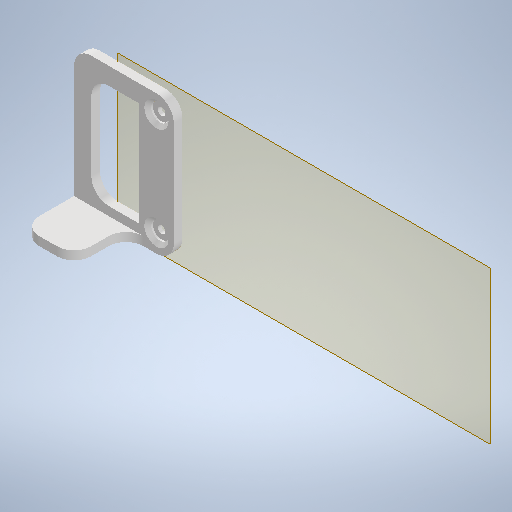
# Autodesk Inventor part: led 7 seg v3_stand
Saved by Autodesk Inventor 2026 (Build 300175000, 175)
## iProperties
Created: 2025-07-07
Part Number: led 7 seg v3_stand
Material: Generic
Document SubType Name: Modeling
Designer: Korobeynikov
Density: 1 g/cm^3
Appearance: Default
Author: Korobeynikov
Autodesk Inventor part; units mm, degrees
ref_plane "YZ Plane" through (0, 0, 0) normal (1, 0, 0) x (0, 1, 0)
ref_plane "XZ Plane" through (0, 0, 0) normal (0, 1, 0) x (-1, 0, 0)
ref_plane "XY Plane" through (0, 0, 0) normal (0, 0, 1) x (1, 0, 0)
ref_plane "Work Plane1" through (0, 0, 0) normal (0, 0, 1) x (1, 0, 0)
sketch "Sketch1" plane through (0, 0, 0) normal (0, 0, 1) x (1, 0, 0)
  circle A0 centre (-80, 29.5) radius 2.15 projected
  circle A1 centre (-80, -29.5) radius 2.15 projected
  line L0 (-127.5, 40) -> (-70, 40)
  line L1 (-70, 40) -> (-70, -40)
  line L2 (-70, -40) -> (-127.5, -40)
  line L3 (-127.5, -40) -> (-127.5, 40)
  line L4 (87.5, 40) -> (-87.5, 40) projected
  line L5 (-87.5, -40) -> (87.5, -40) projected
  line L6 (-97.5, 30) -> (-97.5, -30) projected
  line L7 (-117.5, 30) -> (-90, 30)
  line L8 (-90, 30) -> (-90, -30)
  line L9 (-90, -30) -> (-117.5, -30)
  line L10 (-117.5, -30) -> (-117.5, 30)
  point P0 (0, 0)
  point P1 (-117.5, 0)
  point P2 (-127.5, 0)
  dimension "d0" = 10
  dimension "d1" = 30
  dimension "d2" = 10
  dimension "d3" = 10
  dimension "d4" = 10
  constraints: 16 end point, 4 parallel, 2 horizontal, 2 midpoint, 2 perpendicular, 2 point on line, 1 horizontal alignment
  measures "d0" distance from line of L1 A0.centre
  measures "d1" distance between parallel lines of L3 L6
  measures "d2" distance between parallel lines of L0 L7
  measures "d3" distance between parallel lines of L3 L10
  measures "d4" distance from line of A0.centre L8
extrude "Extrusion1" add sketch "Sketch1" along normal blind 5
sketch "Sketch2" plane through (0, 0, 5) normal (0, 0, 1) x (1, 0, 0)
  line L0 (-127.5, -40) -> (-70, -40) projected
  line L1 (-127.5, -40) -> (-97.5, -40)
  line L2 (-97.5, -40) -> (-97.5, -35)
  line L3 (-97.5, -35) -> (-127.5, -35)
  line L4 (-127.5, -35) -> (-127.5, -40)
  line L5 (-97.5, 30) -> (-97.5, -30) projected
  point P0 (0, 0)
  dimension "d7" = 5
  dimension "d8" = 30
  constraints: 8 end point, 2 parallel, 1 horizontal, 1 perpendicular, 1 point on line
  measures "d7" distance of L1.end L2.end
  measures "d8" distance of L2.end L3.end
extrude "Extrusion2" add sketch "Sketch2" along normal blind 30
sketch "Sketch3" plane through (0, 0, 5) normal (0, 0, 1) x (1, 0, 0)
  circle A0 centre (-80, 29.5) radius 2.15 projected
  circle A1 centre (-80, 29.5) radius 5
  circle A2 centre (-80, -29.5) radius 2.15 projected
  circle A3 centre (-80, -29.5) radius 5
  point P0 (0, 0)
  dimension "d11" = 10
  dimension "d12" = 10
  constraints: 2 centre point, 2 coincident
  measures "d11" diameter of A1
  measures "d12" diameter of A3
extrude "Extrusion3" cut sketch "Sketch3" against normal blind 3
chamfer "Chamfer1" distance 2 angle 45 2 edges at (-85, 29.5, 5) (-85, -29.5, 5)
fillet "Fillet1" radius 10 3 edges at (-127.5, -37.5, 35) (-97.5, -37.5, 35) (-97.5, -37.5, 5)
fillet "Fillet2" radius 10 5 edges at (-127.5, 40, 2.5) (-117.5, 30, 2.5) (-117.5, -30, 2.5) (-70, 40, 2.5) (-70, -40, 2.5)
body "Solid1"
